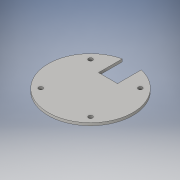
# Autodesk Inventor part: LiDAR_mount_spacer_Rev.1
Saved by Autodesk Inventor 2016 (Build 200138000, 138)
## iProperties
Created: 2018-03-09
Part Number: LiDAR_mount_spacer_Rev.1
Material: Aluminum 6061
Document SubType Name: Modeling
Designer: emvanzant
Density: 2.7 g/cm^3
Appearance: Aluminum - Flat
Author: emvanzant
Autodesk Inventor part; units mm, degrees
ref_plane "YZ Plane" through (0, 0, 0) normal (1, 0, 0) x (0, 1, 0)
ref_plane "XZ Plane" through (0, 0, 0) normal (0, 1, 0) x (-1, 0, 0)
ref_plane "XY Plane" through (0, 0, 0) normal (0, 0, 1) x (1, 0, 0)
sketch "Sketch2" plane through (0, 0, 0) normal (0, 1, 0) x (-1, 0, 0)
  arc A0 (5.75, -24.8433) -> (-5.75, -24.8433) centre (0, 0) ccw
  line L0 (-5.75, -24.8433) -> (5.75, -24.8433)
  line L1 (5.75, -24.8433) -> (5.75, -10.5)
  line L2 (5.75, -10.5) -> (-5.75, -10.5)
  line L3 (-5.75, -10.5) -> (-5.75, -24.8433)
  line L4 (-15, 15) -> (15, 15) construction
  line L5 (15, 15) -> (15, -15) construction
  line L6 (15, -15) -> (-15, -15) construction
  line L7 (-15, -15) -> (-15, 15) construction
  line L8 (-15, 15) -> (15, -15) construction
  line L9 (15, 15) -> (-15, -15) construction
  dimension "d1" = 51
  dimension "d2" = 10.5
  dimension "d3" = 11.5
  dimension "d4" = 30
  dimension "d5" = 30
  constraints: 20 end point, 5 coincident, 4 parallel, 2 horizontal, 2 midpoint, 2 perpendicular, 2 point on circle, 1 centre point
  measures "d1" diameter of A0
  measures "d2" distance from line of L2 point (0, 0)
  measures "d3" distance of L1.end L2.end
  measures "d4" distance of L5.end L6.end
  measures "d5" distance of L4.end L5.end
extrude "Extrusion1" add sketch "Sketch2" along normal blind 1.5875 contours L1 L2 L3 A0
hole "Hole1" at (15, 0, -15) at (-15, 0, -15) at (-15, 0, 15) at (15, 0, 15) direction (0, 1, 0) diameter 2.5 end through all
body "Solid1"
